Autodesk Inventor part; units mm, degrees
(part 2 of 2)
  spline S239 degree 2 poles (-56.2892, 197.3924) (-56.2494, 197.435) (-56.1815, 197.4223) knots 0 0 0 1 1 1
  spline S240 degree 2 poles (-56.1815, 197.4223) (-56.1325, 197.4127) (-56.0609, 197.3458) knots 0 0 0 1 1 1
  line L231 (-56.0609, 197.3458) -> (-56.0048, 197.2933)
  line L232 (-56.0048, 197.2933) -> (-55.2757, 196.6117)
  line L233 (-55.2757, 196.6117) -> (-55.2331, 196.572)
  spline S241 degree 2 poles (-55.2331, 196.572) (-55.1751, 196.5177) (-55.1529, 196.4136) (-55.1908, 196.3729) knots 0 0 0 1 2 2 2
  spline S242 degree 2 poles (-55.1908, 196.3729) (-55.2523, 196.3072) (-55.338, 196.3474) knots 0 0 0 1 1 1
  spline S243 degree 2 poles (-55.338, 196.3474) (-55.4102, 196.3787) (-55.4348, 196.3872) (-55.459, 196.3808) knots 0 0 0 1 2 2 2
  spline S244 degree 2 poles (-55.459, 196.3808) (-55.5018, 196.3737) (-55.5561, 196.3157) knots 0 0 0 1 1 1
  line L234 (-55.5561, 196.3157) -> (-57.082, 194.6833)
  spline S245 degree 2 poles (-57.082, 194.6833) (-57.1362, 194.6253) (-57.1404, 194.5821) knots 0 0 0 1 1 1
  spline S246 degree 2 poles (-57.1404, 194.5821) (-57.1452, 194.5575) (-57.135, 194.5335) (-57.0971, 194.4655) knots 0 0 0 1 2 2 2
  spline S247 degree 2 poles (-57.0971, 194.4655) (-57.0513, 194.3828) (-57.1146, 194.3151) knots 0 0 0 1 1 1
  spline S248 degree 2 poles (-57.1146, 194.3151) (-57.1525, 194.2744) (-57.2579, 194.2896) (-57.316, 194.3439) knots 0 0 0 1 2 2 2
  line L235 (-57.316, 194.3439) -> (-57.3585, 194.3836)
  line L236 (-57.3585, 194.3836) -> (-58.0857, 195.0635)
  spline S249 degree 2 poles (-57.5236, 196.669) (-57.6526, 196.8295) (-57.7626, 197.0374) (-57.7832, 197.1473) knots 0 0 0 1 2 2 2
  spline S250 degree 2 poles (-57.7832, 197.1473) (-57.8039, 197.2608) (-57.7472, 197.4688) (-57.6731, 197.5481) knots 0 0 0 1 2 2 2
  line L237 (-57.6731, 197.5481) -> (-57.3585, 197.8846)
  spline S251 degree 2 poles (-57.3585, 197.8846) (-57.3078, 197.9388) (-57.3427, 197.9713) knots 0 0 0 1 1 1
  spline S252 degree 2 poles (-57.3427, 197.9713) (-57.3543, 197.9822) (-57.3881, 197.9848) (-57.4234, 197.978) knots 0 0 0 1 2 2 2
  spline S253 degree 2 poles (-57.4234, 197.978) (-57.5165, 197.9598) (-57.559, 197.9996) knots 0 0 0 1 1 1
  spline S254 degree 2 poles (-57.559, 197.9996) (-57.5861, 198.0249) (-57.588, 198.1354) (-57.559, 198.1663) knots 0 0 0 1 2 2 2
  spline S255 degree 2 poles (-57.559, 198.1663) (-57.512, 198.2166) (-57.2797, 198.2713) (-57.1539, 198.2624) knots 0 0 0 1 2 2 2
  spline S256 degree 2 poles (-57.1539, 198.2624) (-57.0393, 198.2531) (-56.8375, 198.155) (-56.7311, 198.0556) knots 0 0 0 1 2 2 2
  spline S257 degree 2 poles (-56.7311, 198.0556) (-56.5164, 197.8549) (-56.5061, 197.3814) (-56.7104, 197.1628) knots 0 0 0 1 2 2 2
  line L238 (-56.7104, 197.1628) -> (-56.9671, 196.8882)
  spline S258 degree 2 poles (-56.9671, 196.8882) (-57.0521, 196.7973) (-57.0646, 196.78) knots 0 0 0 1 1 1
  spline S259 degree 2 poles (-57.0646, 196.78) (-57.1184, 196.707) (-57.1231, 196.6244) knots 0 0 0 1 1 1
  spline S260 degree 2 poles (-57.1231, 196.6244) (-57.1309, 196.523) (-57.051, 196.4301) knots 0 0 0 1 1 1
  line L239 (-57.051, 196.4301) -> (-57.2137, 196.2561)
  spline S261 degree 2 poles (-57.2137, 196.2561) (-57.3153, 196.3257) (-57.3828, 196.3272) knots 0 0 0 1 1 1
  spline S262 degree 2 poles (-57.3828, 196.3272) (-57.4428, 196.3289) (-57.5384, 196.277) (-57.6071, 196.2035) knots 0 0 0 1 2 2 2
  line L240 (-57.6071, 196.2035) -> (-58.0121, 195.7702)
  spline S263 degree 2 poles (-58.0121, 195.7702) (-58.108, 195.6677) (-58.1227, 195.493) (-58.0454, 195.3664) knots 0 0 0 1 2 2 2
  line L241 (-58.0454, 195.3664) -> (-58.2153, 195.1846)
  line L242 (-58.2153, 195.1846) -> (-58.2579, 195.2244)
  spline S264 degree 2 poles (-58.2579, 195.2244) (-58.4377, 195.3925) (-58.5527, 195.5254) knots 0 0 0 1 1 1
  spline S265 degree 2 poles (-58.5527, 195.5254) (-58.726, 195.72) (-58.7755, 195.9656) knots 0 0 0 1 1 1
  spline S266 degree 2 poles (-58.7755, 195.9656) (-58.8472, 196.3153) (-58.5832, 196.5977) knots 0 0 0 1 1 1
  spline S267 degree 2 poles (-58.5832, 196.5977) (-58.3681, 196.8278) (-58.0876, 196.841) knots 0 0 0 1 1 1
  spline S268 degree 2 poles (-58.0876, 196.841) (-57.9697, 196.8469) (-57.735, 196.7724) (-57.5236, 196.669) knots 0 0 0 1 2 2 2
  constraints: 2 other
extrude "Extrusion4" cut sketch "Sketch4" against normal through all contours L76 L77 L78 S0 S1 S2 L79 S3 S4 S5 S6 S7 L80 | L81 L82 L83 L84 L85 L86 | L87 L88 S8 S9 S10 S11 L89 S12 S13 S14 S15 L90 | L91 L92 S16 S17 S18 S19 L93 S20 S21 S22 S23 L94 L95 L96 L97 L98 L99 | L100 L101 S24 S25 L102 S26 S27 L103 S28 S29 S30 S31 L104 | L105 S32 S33 S34 S35 S36 L106 L107 L108 S37 S38 S39 S40 L109 S41 S42 S43 S44 L110 L111 | S45 S46 L112 S47 S48 S49 S50 S51 S52 S53 L113 S54 S55 S56 L114 S57 S58 L115 S59 L116 L117 S60 S61 S62 S63 S64 | L118 L119 L120 L121 S65 L122 S66 S67 S68 L123 | L124 L125 S69 L126 S70 S71 S72 L127 S73 S74 S75 L128 | L129 L130 S76 S77 S78 L131 S79 S80 S81 S82 S83 L132 | L133 L134 S84 S85 S86 S87 L135 S88 S89 S90 S91 L136 L137 L138 S92 S93 S94 S95 L139 S96 S97 S98 S99 L140 | L141 L142 L143 L144 S100 L145 S101 S102 S103 L146 | L147 L148 S104 L149 S105 S106 S107 L150 S108 S109 S110 L151 | L152 L153 S111 S112 S113 L154 S114 S115 S116 S117 S118 L155 | L156 S119 L157 S120 S121 L158 S122 S123 S124 S125 S126 S127 | S128 S129 L159 S130 S131 L160 S132 S133 S134 S135 L161 L162 S136 S137 S138 L163 | L164 S139 S140 S141 S142 S143 L165 S144 S145 S146 S147 | L166 L167 L168 S148 S149 S150 S151 L169 S152 S153 S154 S155 L170 L171 | S156 S157 S158 S159 L172 L173 S160 S161 L174 S162 S163 L175 S164 S165 L176 L177 S166 S167 L178 L179 S168 S169 S170 S171 | L180 S172 S173 S174 S175 L181 L182 L183 L184 S176 S177 S178 S179 L185 S180 S181 L186 L187 S182 S183 S184 | L188 S185 S186 L189 S187 S188 S189 L190 S190 S191 S192 S193 S194 L191 S195 S196 S197 | L192 L193 L194 L195 L196 L197 | L198 L199 S198 S199 S200 S201 L200 | L201 L202 S202 S203 S204 S205 L203 | L204 L205 L206 L207 L208 L209 | L210 L211 S206 S207 S208 S209 L212 | L213 L214 S210 S211 S212 S213 L215 | L216 L217 L218 S214 S215 S216 S217 L219 S218 S219 S220 S221 L220 L221 | L222 S222 S223 S224 S225 L223 L224 | L225 L226 S226 S227 S228 L227 | L228 S229 S230 S231 S232 L229 S233 S234 S235 | L230 S236 S237 S238 S239 S240 L231 L232 L233 S241 S242 S243 S244 L234 S245 S246 S247 S248 L235 L236 | S249 S250 L237 S251 S252 S253 S254 S255 S256 S257 L238 S258 S259 S260 L239 S261 S262 L240 S263 L241 L242 S264 S265 S266 S267 S268
body "Solid1"
